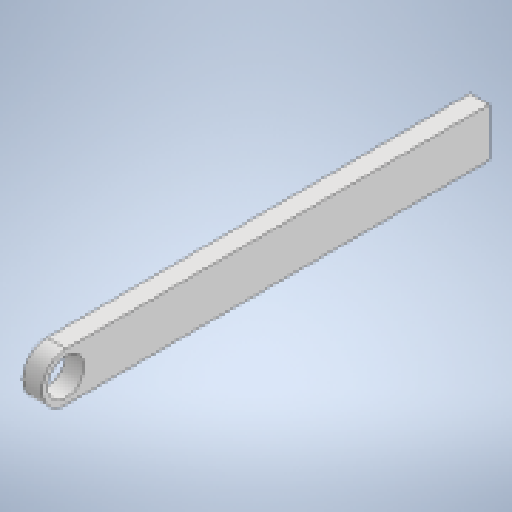
# Autodesk Inventor part: wach
Saved by Autodesk Inventor 2023 (Build 270158000, 158)
## iProperties
Created: 2023-07-30
Part Number: wach
Material: Ogólny
Document SubType Name: Modeling
Designer: Kamil
Density: 1 g/cm^3
Appearance: Domyślna
Author: Kamil
Autodesk Inventor part; units mm, degrees
ref_plane "YZ Plane" through (0, 0, 0) normal (1, 0, 0) x (0, 1, 0)
ref_plane "XZ Plane" through (0, 0, 0) normal (0, 1, 0) x (-1, 0, 0)
ref_plane "XY Plane" through (0, 0, 0) normal (0, 0, 1) x (1, 0, 0)
sketch "Szkic1" plane through (0, 0, 0) normal (1, 0, 0) x (0, 1, 0)
  circle A0 centre (0, 0) radius 1.9
  circle A1 centre (0, 0) radius 2.5
  line L0 (2.5, 0) -> (-2.5, 0)
  line L1 (-2.5, 0) -> (-2.5, -45)
  line L2 (-2.5, -45) -> (2.5, -45)
  line L3 (2.5, -45) -> (2.5, 0)
  dimension "d1" = 5
  dimension "d0" = 3.8
  dimension "d2" = 45
  constraints: 8 end point, 2 coincident, 2 parallel, 1 centre point, 1 horizontal, 1 perpendicular, 3 other
  measures "d0" diameter of A0
  measures "d2" distance of L1.end L0.end
extrude "Wyciągnięcie proste1" add sketch "Szkic1" along normal blind 2 contours L0 A1 A0 | A0 L0 A1 | L3 L2 L1 A1
sketch "Szkic2" plane through (0, -2.5, -45) normal (0, 0, -1) x (-1, 0, 0)
  line L0 (0, 0) -> (0, 5) projected
  line L1 (0, 5) -> (-2, 5) projected
  line L2 (-2, 0) -> (-2, 5) projected
  line L3 (0, 0) -> (-2, 0) projected
  point P0 (0, 2.5)
extrude "Wyciągnięcie proste2" cut sketch "Szkic2" against normal blind 1.125
